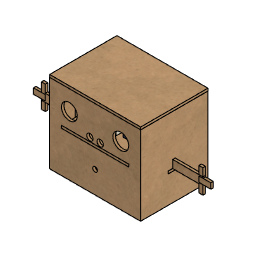
CAD final (Autodesk Fusion 360 design; units mm, degrees)
Autodesk Fusion 360 part; units mm, degrees
sketch "Sketch1" plane through (0, 0, 0) normal (0, 0, 1) x (1, 0, 0)
  line L0 (-32.3795, 47.4843) -> (40, 47.4843)
  line L1 (40, 47.4843) -> (40, -5)
  line L2 (40, -5) -> (-32.3795, -5)
  line L3 (-32.3795, -5) -> (-32.3795, 47.4843)
  constraint horizontal L0
  constraint vertical L1
  constraint horizontal L2
  constraint vertical L3
sketch "Sketch2" plane through (0, 0, 0) normal (0, 0, 1) x (1, 0, 0)
sketch "Sketch3" plane through (0, 0, 0) normal (0, 0, 1) x (1, 0, 0)
  line L0 (-70, 30) -> (-16.7, 30)
  line L1 (-16.7, 30) -> (-16.7, -38.6)
  line L2 (-16.7, -38.6) -> (-70, -38.6)
  line L3 (-70, -38.6) -> (-70, 30)
  dimension "d3" = 53.3
  dimension "d4" = 68.6
  constraint horizontal L0
  constraint vertical L1
  constraint horizontal L2
  constraint vertical L3
  measures "d3" distance of L0.start L0.end
  measures "d4" distance of L0.start L2.end
extrude "Extrude2" add sketch "Sketch3" along normal blind 10 makes body 1
move_body "Move3" bodies 1 to x (0, -1, 0) y (1, 0, 0) z (0, 0, 1) at (-31.4, -108.6, 0)
move_body "Move4" bodies 1 to x (1, 0, 0) y (0, 1, 0) z (0, 0, 1) at (-5.9347, 58.8273, -1.6422)
sketch "Sketch4" plane through (0, 0, 0) normal (0, 0, 1) x (1, 0, 0)
  line L0 (40, 25) -> (125, 25)
  line L1 (125, 25) -> (125, -30)
  line L2 (125, -30) -> (40, -30)
  line L3 (40, -30) -> (40, 25)
  dimension "d7" = 85
  dimension "d8" = 55
  constraint horizontal L0
  constraint vertical L1
  constraint horizontal L2
  constraint vertical L3
  measures "d7" distance of L0.start L0.end
  measures "d8" distance of L0.start L2.end
extrude "Extrude3" add sketch "Sketch4" along normal blind 10 separate body makes body 2
move_body "Move5" bodies 1 to x (0, 1, 0) y (-1, 0, 0) z (0, 0, 1) at (-109.0073, 42.862, 0)
move_body "Move6" bodies 1 to x (1, 0, 0) y (0, 1, 0) z (0, 0, 1) at (69.2901, 3.0727, 11.6422)
move_body "Move7" bodies 2 to x (0, 1, 0) y (-1, 0, 0) z (0, 0, 1) at (10, -70, 0)
move_body "Move8" bodies 2 to x (1, 0, 0) y (0, 1, 0) z (0, 0, 1) at (13.4816, 0.9657, 8.7354)
sketch "Sketch5" plane through (0, 0, 0) normal (0, 0, 1) x (1, 0, 0)
  line L0 (100, -150) -> (-130, -150)
  line L1 (-130, -150) -> (-130, 20)
  line L2 (-130, 20) -> (100, 20)
  line L3 (100, 20) -> (100, -150)
  dimension "d11" = 230
  dimension "d12" = 170
  constraint horizontal L0
  constraint vertical L1
  constraint horizontal L2
  constraint vertical L3
  measures "d11" distance of L0.start L0.end
  measures "d12" distance of L0.start L2.end
extrude "Extrude4" add sketch "Sketch5" against normal blind 200 separate body makes body 3
sketch "Sketch6" plane through (0, 0, -200) normal (0, 0, -1) x (1, 0, 0)
  line L0 (-130, -20) -> (100, -20)
  line L1 (100, -20) -> (100, 150)
  line L2 (100, 150) -> (-130, 150)
  line L3 (-130, 150) -> (-130, -20)
  line L4 (-122.8889, 140.963) -> (94.4111, 140.963)
  line L5 (94.4111, 140.963) -> (94.4111, -12.737)
  line L6 (94.4111, -12.737) -> (-122.8889, -12.737)
  line L7 (-122.8889, -12.737) -> (-122.8889, 140.963)
  dimension "d15" = 217.3
  dimension "d16" = 153.7
  constraint horizontal L4
  constraint vertical L5
  constraint horizontal L6
  constraint vertical L7
  measures "d15" distance of L4.start L4.end
  measures "d16" distance of L4.start L6.end
extrude "Extrude5" cut sketch "Sketch6" against normal blind 193.35 contours L4 L5 L6 L7 bodies 3
move_body "Move9" bodies 1 to x (1, 0, 0) y (0, 1, 0) z (0, 0, 1) at (-192.1553, -38.6436, -133.7239)
move_body "Move10" bodies 2 to x (1, 0, 0) y (0, 1, 0) z (0, 0, 1) at (-190.1426, -42.9302, -139.0807)
sketch "Sketch7" plane through (0, 0, 0) normal (0, 0, 1) x (1, 0, 0)
  line L0 (-116.7221, 87.5547) -> (113.2779, 87.5547)
  line L1 (113.2779, 87.5547) -> (113.2779, 257.5547)
  line L2 (113.2779, 257.5547) -> (-116.7221, 257.5547)
  line L3 (-116.7221, 257.5547) -> (-116.7221, 87.5547)
  dimension "d19" = 230
  dimension "d20" = 170
  constraint horizontal L0
  constraint vertical L1
  constraint horizontal L2
  constraint vertical L3
  measures "d19" distance of L0.start L0.end
  measures "d20" distance of L0.start L2.end
extrude "Extrude6" add sketch "Sketch7" along normal blind 6.35 separate body makes body 4
move_body "Move11" bodies 4 to x (1, 0, 0) y (0, 1, 0) z (0, 0, 1) at (-13.2084, -237.8923, -206.1761)
sketch "Sketch8" plane through (0, 20, 0) normal (0, 1, 0) x (-1, 0, 0)
  line L0 (130, 0) -> (-100, 0)
  line L1 (-100, 0) -> (-100, -200)
  line L2 (-100, -200) -> (130, -200)
  line L3 (130, -200) -> (130, 0)
  line L4 (100, -110) -> (-72.7396, -110)
  line L5 (-72.7396, -110) -> (-72.7396, -103.65)
  line L6 (-72.7396, -103.65) -> (100, -103.65)
  line L7 (100, -103.65) -> (100, -110)
  dimension "d23" = 6.35
  constraint horizontal L4
  constraint vertical L5
  constraint horizontal L6
  constraint vertical L7
  measures "d23" distance of L4.start L6.end
extrude "Extrude7" cut sketch "Sketch8" against normal blind 200 contours L4 L5 L6 L7 bodies 3
sketch "Sketch9" plane through (0, 0, 0) normal (0, 0, 1) x (1, 0, 0)
  line L0 (-120, 110) -> (52.74, 110)
  line L1 (52.74, 110) -> (52.74, 280)
  line L2 (52.74, 280) -> (-120, 280)
  line L3 (-120, 280) -> (-120, 110)
  dimension "d26" = 172.74
  dimension "d27" = 170
  constraint horizontal L0
  constraint vertical L1
  constraint horizontal L2
  constraint vertical L3
  measures "d26" distance of L0.start L0.end
  measures "d27" distance of L0.start L2.end
extrude "Extrude8" add sketch "Sketch9" against normal blind 6.35 separate body makes body 5
move_body "Move12" bodies 5 to x (1, 0, 0) y (0, 1, 0) z (0, 0, 1) at (20.107, -259.5032, -103.2368)
sketch "Sketch10" plane through (0, -150, 0) normal (0, -1, 0) x (1, 0, 0)
  line L0 (72.7396, -103.65) -> (72.7396, -110)
  line L1 (72.7396, -110) -> (-100, -110)
  line L2 (-100, -110) -> (-100, -103.65)
  line L3 (-100, -103.65) -> (72.7396, -103.65)
  line L4 (100, 0) -> (-130, 0)
  line L5 (-130, 0) -> (-130, -200)
  line L6 (-130, -200) -> (100, -200)
  line L7 (100, -200) -> (100, 0)
  circle A0 centre (50, -150) radius 20
  circle A1 centre (50, -150) radius 20
  circle A2 centre (-80, -150) radius 20
extrude "Extrude9" cut sketch "Sketch10" against normal blind 20 contours A0 A1 | A2 bodies 3
sketch "Sketch11" plane through (0, -150, 0) normal (0, -1, 0) x (1, 0, 0)
  circle A0 centre (-80, -150) radius 20
  circle A1 centre (50, -150) radius 20
  line L0 (72.7396, -103.65) -> (72.7396, -110)
  line L1 (72.7396, -110) -> (-100, -110)
  line L2 (-100, -110) -> (-100, -103.65)
  line L3 (-100, -103.65) -> (72.7396, -103.65)
  line L4 (100, 0) -> (-130, 0)
  line L5 (-130, 0) -> (-130, -200)
  line L6 (-130, -200) -> (100, -200)
  line L7 (100, -200) -> (100, 0)
  circle A2 centre (-1.9497, -120.0498) radius 8.05
  dimension "d32" = 16.1
  measures "d32" diameter of A2
sketch "Sketch12" plane through (0, -150, 0) normal (0, -1, 0) x (1, 0, 0)
sketch "Sketch13" plane through (0, -150, 0) normal (0, -1, 0) x (1, 0, 0)
  circle A0 centre (-28.05, -120.05) radius 8.05
  dimension "d33" = 16.1
  measures "d33" diameter of A0
extrude "Extrude10" cut sketch "Sketch11" sketch "Sketch13" against normal blind 10 contours A2 of sketch 2 bodies 3
move_body "Move13" bodies 4 to x (1, 0, 0) y (0, 1, 0) z (0, 0, 1) at (231.7541, -19.2478, 6.1761)
move_body "Move14" bodies 2 to x (1, 0, 0) y (0, 1, 0) z (0, 0, 1) at (189.899, -32.0286, 10.5679)
move_body "Move15" bodies 1 to x (1, 0, 0) y (0, 1, 0) z (0, 0, 1) at (183.6878, -30.6758, -12.2886)
move_body "Move16" bodies 1 to x (1, 0, 0) y (0, 1, 0) z (0, 0, 1) at (0, 0, 15)
sketch "Sketch14" plane through (100, 0, 0) normal (1, 0, 0) x (0, 1, 0)
sketch "Sketch15" plane through (100, 0, 0) normal (1, 0, 0) x (0, 1, 0)
  line L0 (-50, -75) -> (-80, -75)
  line L1 (-80, -75) -> (-80, -68.65)
  line L2 (-80, -68.65) -> (-50, -68.65)
  line L3 (-50, -68.65) -> (-50, -75)
  dimension "d36" = 6.35
  constraint horizontal L0
  constraint vertical L1
  constraint horizontal L2
  constraint vertical L3
  measures "d36" distance of L0.start L2.end
extrude "Extrude11" cut sketch "Sketch15" against normal blind 320 bodies 3
sketch "Sketch16" plane through (0, 0, 0) normal (0, 0, 1) x (1, 0, 0)
  line L0 (-100, 140) -> (130, 140)
  line L1 (130, 140) -> (130, 170)
  line L2 (130, 170) -> (-100, 170)
  line L3 (-100, 170) -> (-100, 140)
  dimension "d39" = 230
  dimension "d40" = 30
  constraint horizontal L0
  constraint vertical L1
  constraint horizontal L2
  constraint vertical L3
  measures "d39" distance of L0.start L0.end
  measures "d40" distance of L0.start L2.end
extrude "Extrude12" add sketch "Sketch16" against normal blind 6.35 separate body makes body 6
move_body "Move17" bodies 6 to x (1, 0, 0) y (0, 1, 0) z (0, 0, 1) at (-29.7399, -217.8653, -68.3754)
move_body "Move18" bodies 6 to x (1, 0, 0) y (0, 1, 0) z (0, 0, 1) at (0, -2.152, 0)
sketch "Sketch17" plane through (0, 0, -74.7254) normal (0, 0, -1) x (1, 0, 0)
  line L0 (-129.7399, 80.0173) -> (-129.7399, 50.0173)
  line L1 (-129.7399, 50.0173) -> (100.2601, 50.0173)
  line L2 (100.2601, 50.0173) -> (100.2601, 80.0173)
  line L3 (100.2601, 80.0173) -> (-129.7399, 80.0173)
sketch "Sketch18" plane through (0, 0, -74.7254) normal (0, 0, -1) x (1, 0, 0)
  line L0 (90.26, 76.717) -> (86.61, 76.717)
  line L1 (86.61, 76.717) -> (86.61, 64.717)
  line L2 (86.61, 64.717) -> (90.26, 64.717)
  line L3 (90.26, 64.717) -> (90.26, 76.717)
  dimension "d43" = 3.65
  constraint horizontal L0
  constraint vertical L1
  constraint horizontal L2
  constraint vertical L3
  measures "d43" distance of L0.start L0.end
sketch "Sketch19" plane through (0, 0, -74.7254) normal (0, 0, -1) x (1, 0, 0)
  line L0 (60.61, 64.717) -> (56.96, 64.717)
  line L1 (56.96, 64.717) -> (56.96, 76.717)
  line L2 (56.96, 76.717) -> (60.61, 76.717)
  line L3 (60.61, 76.717) -> (60.61, 64.717)
  dimension "d44" = 3.65
  constraint horizontal L0
  constraint vertical L1
  constraint horizontal L2
  constraint vertical L3
  measures "d44" distance of L0.start L0.end
extrude "Extrude13" cut sketch "Sketch18" against normal blind 11 bodies 6
extrude "Extrude14" cut sketch "Sketch19" against normal blind 22 bodies 6
sketch "Sketch20" plane through (0, 0, 0) normal (0, 0, 1) x (1, 0, 0)
  line L0 (95, -105) -> (91.35, -105)
  line L1 (91.35, -105) -> (91.35, -117)
  line L2 (91.35, -117) -> (95, -117)
  line L3 (95, -117) -> (95, -105)
  dimension "d49" = 3.65
  dimension "d50" = 12
  constraint horizontal L0
  constraint vertical L1
  constraint horizontal L2
  constraint vertical L3
  measures "d49" distance of L0.start L0.end
  measures "d50" distance of L0.start L2.end
sketch "Sketch21" plane through (0, 0, 0) normal (0, 0, 1) x (1, 0, 0)
  line L0 (65.35, -105) -> (61.7, -105)
  line L1 (61.7, -105) -> (61.7, -117)
  line L2 (61.7, -117) -> (65.35, -117)
  line L3 (65.35, -117) -> (65.35, -105)
  dimension "d51" = 3.65
  dimension "d52" = 12
  constraint horizontal L0
  constraint vertical L1
  constraint horizontal L2
  constraint vertical L3
  measures "d51" distance of L0.start L0.end
  measures "d52" distance of L0.start L2.end
extrude "Extrude15" add sketch "Sketch21" against normal blind 25 separate body makes body 7
extrude "Extrude16" add sketch "Sketch20" against normal blind 25 separate body makes body 8
extrude "Extrude17" cut 1 faces at (86.61, -72.717, -72.6087) along direction (-1, 0, 0) blind 2.65 on bodies 6 bodies 6
extrude "Extrude18" cut 1 faces at (83.96, -72.717, -72.6087) along direction (-1, 0, 0) blind 0.05 on bodies 6 bodies 6
extrude "Extrude19" cut 1 faces at (56.96, -68.717, -72.6087) along direction (-1, 0, 0) blind 6.35 on bodies 6 bodies 6
extrude "Extrude20" add 1 faces at (60.61, -72.717, -72.6087) along direction (-1, 0, 0) blind 3.3 on bodies 6 bodies 6
extrude "Extrude21" cut 1 faces at (57.31, -72.717, -72.6087) along direction (1, 0, 0) blind 0.6 on bodies 6 bodies 6
extrude "Extrude22" add 1 faces at (50.61, -68.717, -72.6087) along direction (1, 0, 0) blind 0.95 on bodies 6 bodies 6
extrude "Extrude23" add 1 faces at (91.35, -109, -8.3333) along direction (-1, 0, 0) blind 0.7 on bodies 8 bodies 8
extrude "Extrude24" cut 1 faces at (65.35, -113, -8.3333) along direction (-1, 0, 0) blind 0.7 on bodies 7 bodies 7
extrude "Extrude25" add 1 faces at (61.7, -109, -8.3333) along direction (-1, 0, 0) blind 1.4 on bodies 7 bodies 7
extrude "Extrude26" add 1 faces at (90.65, -109, -8.3333) along direction (-1, 0, 0) blind 2 on bodies 8 bodies 8
extrude "Extrude27" cut 1 faces at (64.65, -113, -8.3333) along direction (-1, 0, 0) blind 2 on bodies 7 bodies 7
extrude "Extrude28" add 1 faces at (60.3, -109, -8.3333) along direction (-1, 0, 0) blind 4 on bodies 7 bodies 7
sketch "Sketch22" plane through (56.3, 0, 0) normal (-1, 0, 0) x (0, -1, 0)
extrude "Extrude29" cut 1 faces at (86.0267, -64.717, -70.4921) along direction (0, 1, 0) blind 10 on bodies 6 bodies 6
extrude "Extrude30" cut 1 faces at (53.6767, -64.717, -70.4921) along direction (0, 1, 0) blind 10 on bodies 6 bodies 6
extrude "Extrude31" add 1 faces at (60.5333, -105, -8.3333) along direction (0, 1, 0) blind 10 on bodies 7 bodies 7
extrude "Extrude32" add 1 faces at (92.8833, -105, -8.3333) along direction (0, 1, 0) blind 10 on bodies 8 bodies 8
sketch "Sketch23" plane through (56.3, 0, 0) normal (-1, 0, 0) x (0, -1, 0)
  line L0 (113.4998, -12.7498) -> (98.4998, -12.7498)
  line L1 (98.4998, -12.7498) -> (98.4998, -6.3998)
  line L2 (98.4998, -6.3998) -> (113.4998, -6.3998)
  line L3 (113.4998, -6.3998) -> (113.4998, -12.7498)
  dimension "d91" = 15
  dimension "d92" = 6.35
  constraint horizontal L0
  constraint vertical L1
  constraint horizontal L2
  constraint vertical L3
  measures "d91" distance of L0.start L0.end
  measures "d92" distance of L0.start L2.end
extrude "Extrude33" add 1 faces at (60.5333, -109.6667, -25) along direction (0, 0, -1) blind 5.85 on bodies 7 bodies 7
extrude "Extrude34" add 1 faces at (90.7667, -102.3333, -25) along direction (0, 0, -1) blind 5.85 on bodies 8 bodies 8
sketch "Sketch24" plane through (56.3, 0, 0) normal (-1, 0, 0) x (0, -1, 0)
  line L0 (95, -30.85) -> (117, -30.85)
  line L1 (113.5, -31) -> (98.5, -31)
  line L2 (98.5, -31) -> (98.5, -24.65)
  line L3 (98.5, -24.65) -> (113.5, -24.65)
  line L4 (113.5, -24.65) -> (113.5, -31)
  dimension "d97" = 15
  dimension "d98" = 6.35
  constraint horizontal L1
  constraint vertical L2
  constraint horizontal L3
  constraint vertical L4
  measures "d97" distance of L1.start L1.end
  measures "d98" distance of L1.start L3.end
extrude "Extrude35" add 1 faces at (60.5333, -109.6667, -30.85) along direction (0, 0, -1) blind 3 on bodies 7 bodies 7
extrude "Extrude36" add 1 faces at (90.7667, -102.3333, -30.85) along direction (0, 0, -1) blind 3 on bodies 8 bodies 8
extrude "Extrude37" cut sketch "Sketch24" against normal blind 41 contours L0 L2 L3 L4 bodies 7 8
extrude "Extrude38" cut sketch "Sketch23" against normal blind 39 bodies 7 8
sketch "Sketch25" plane through (0, 0, 0) normal (0, 0, 1) x (1, 0, 0)
  line L0 (55, -135) -> (93.7, -135)
  line L1 (93.7, -135) -> (93.7, -150)
  line L2 (93.7, -150) -> (55, -150)
  line L3 (55, -150) -> (55, -135)
  dimension "d107" = 38.7
  constraint horizontal L0
  constraint vertical L1
  constraint horizontal L2
  constraint vertical L3
  measures "d107" distance of L0.start L0.end
extrude "Extrude39" add sketch "Sketch25" along normal blind 6.35 separate body makes body 9
move_body "Move19" bodies 9 to x (1, 0, 0) y (0, 1, 0) z (0, 0, 1) at (1.3032, 36.5589, -12.7529)
sketch "Sketch26" plane through (0, 0, 0) normal (0, 0, 1) x (1, 0, 0)
  line L0 (-30, 12) -> (8.7, 12)
  line L1 (8.7, 12) -> (8.7, -3)
  line L2 (8.7, -3) -> (-30, -3)
  line L3 (-30, -3) -> (-30, 12)
  dimension "d110" = 38.7
  dimension "d111" = 15
  constraint horizontal L0
  constraint vertical L1
  constraint horizontal L2
  constraint vertical L3
  measures "d110" distance of L0.start L0.end
  measures "d111" distance of L0.start L2.end
extrude "Extrude40" add sketch "Sketch26" along normal blind 6.35 separate body makes body 10
move_body "Move20" bodies 10 to x (1, 0, 0) y (0, 1, 0) z (0, 0, 1) at (86.3471, -110.4772, -31.0644)
move_body "Move21" bodies 7 8 9 10 to x (1, 0, 0) y (0, 1, 0) z (0, 0, 1) at (-4.8384, 40.4721, -68.412)
move_body "Move22" bodies 4 to x (1, 0, 0) y (0, 1, 0) z (0, 0, 1) at (-231.998, 19.5704, 0)
sketch "Sketch27" plane through (94.4111, 0, 0) normal (-1, 0, 0) x (0, -1, 0)
  line L0 (80, -68.65) -> (80, -75)
  line L1 (80, -75) -> (50, -75)
  line L2 (50, -75) -> (50, -68.65)
  line L3 (50, -68.65) -> (80, -68.65)
  line L4 (-12.737, -200) -> (140.963, -200)
  line L5 (140.963, -200) -> (140.963, -6.65)
  line L6 (140.963, -6.65) -> (-12.737, -6.65)
  line L7 (-12.737, -6.65) -> (-12.737, -200)
  line L8 (95, -75) -> (88.65, -75)
  line L9 (88.65, -75) -> (88.65, -111.7682)
  line L10 (88.65, -111.7682) -> (95, -111.7682)
  line L11 (95, -111.7682) -> (95, -75)
  dimension "d114" = 6.35
  constraint horizontal L8
  constraint vertical L9
  constraint horizontal L10
  constraint vertical L11
  measures "d114" distance of L8.start L8.end
extrude "Extrude41" add 1 faces at (72.7396, -143.9753, -107.8833) along direction (-1, 0, 0) blind 2.74 on bodies 3 bodies 3
extrude "Extrude42" cut 1 faces at (72.847, -92.8366, -105.3534) along direction (-1, 0, 0) blind 2.74 on bodies 5 bodies 5
move_body "Move23" bodies 5 to x (1, 0, 0) y (0, 1, 0) z (0, 0, 1) at (0.1843, 0, -0.3685)
extrude "Extrude43" add 1 faces at (72.7396, 17.579, -107.8833) along direction (-1, 0, 0) blind 2.74 on bodies 3 bodies 3
extrude "Extrude44" cut sketch "Sketch27" against normal blind 15 contours L8 L9 L10 L11 bodies 3
extrude "Extrude45" cut 1 faces at (98.137, -90.7667, -111.7682) along direction (0, 0, -1) blind 28 on bodies 3 bodies 3
extrude "Extrude46" cut 1 faces at (96.2741, -95, -118.1788) along direction (0, -1, 0) blind 1.5 on bodies 3 bodies 3
sketch "Sketch28" plane through (0, 0, 0) normal (0, 0, 1) x (1, 0, 0)
  line L0 (60, 60) -> (180, 60)
  line L1 (180, 60) -> (180, 80)
  line L2 (180, 80) -> (60, 80)
  line L3 (60, 80) -> (60, 60)
  constraint horizontal L0
  constraint vertical L1
  constraint horizontal L2
  constraint vertical L3
extrude "Extrude47" add sketch "Sketch28" along normal blind 6.35 separate body makes body 11
extrude "Extrude48" add 1 faces at (94.4111, -8.1753, -93.8833) along direction (-1, 0, 0) blind 0.761 on bodies 3 bodies 3 7 8 9 10 6
extrude "Extrude49" cut 1 faces at (13.5869, -140.963, -38.9833) along direction (0, -1, 0) blind 2.687 on bodies 3 bodies 3
extrude "Extrude50" cut 1 faces at (-122.8889, -70.3043, -158.3333) along direction (-1, 0, 0) blind 0.761 on bodies 3 bodies 3
extrude "Extrude51" cut 1 faces at (13.3333, 12.737, -38.9833) along direction (0, 1, 0) blind 0.913 on bodies 3 bodies 3
sketch "Sketch29" plane through (0, 0, 0) normal (0, 0, 1) x (1, 0, 0)
  line L0 (175, 45) -> (205, 45)
  line L1 (205, 45) -> (205, 55)
  line L2 (205, 55) -> (175, 55)
  line L3 (175, 55) -> (175, 45)
  dimension "d139" = 30
  dimension "d140" = 10
  constraint horizontal L0
  constraint vertical L1
  constraint horizontal L2
  constraint vertical L3
  measures "d139" distance of L0.start L0.end
  measures "d140" distance of L0.start L2.end
extrude "Extrude52" add sketch "Sketch29" along normal blind 6.35 separate body makes body 12
move_body "Move24" bodies 12 to x (0.642788, -0.766044, 0) y (0.766044, 0.642788, 0) z (0, 0, 1) at (20.3326, 165.0215, 1.3134)
move_body "Move25" bodies 12 to x (1, 0, 0) y (0, 1, 0) z (0, 0, 1) at (0, 0, -1)
move_body "Move26" bodies 12 to x (1, 0, 0) y (0, 1, 0) z (0, 0, 1) at (0, 0, -0.31)
move_body "Move27" bodies 12 to x (0.766044, -0.642788, 0) y (0.642788, 0.766044, 0) z (0, 0, 1) at (15.4151, 116.1683, 0)
move_body "Move28" bodies 12 to x (1, 0, 0) y (0, 1, 0) z (0, 0, 1) at (-12, 7, 0)
move_body "Move29" bodies 12 to x (1, 0, 0) y (0, 1, 0) z (0, 0, 1) at (-0.065, 0, 0)
move_body "Move30" bodies 12 to x (1, 0, 0) y (0, 1, 0) z (0, 0, 1) at (0, 8.487, 0)
sketch "Sketch30" plane through (0, 0, 0) normal (0, 0, 1) x (1, 0, 0)
  line L0 (158.5541, 93.3276) -> (188.5541, 93.3276)
  line L1 (188.5541, 93.3276) -> (188.5541, 103.3276)
  line L2 (188.5541, 103.3276) -> (158.5541, 103.3276)
  line L3 (158.5541, 103.3276) -> (158.5541, 93.3276)
  dimension "d143" = 30
  dimension "d144" = 10
  constraint horizontal L0
  constraint vertical L1
  constraint horizontal L2
  constraint vertical L3
  measures "d143" distance of L0.start L0.end
  measures "d144" distance of L0.start L2.end
extrude "Extrude53" add sketch "Sketch30" along normal blind 6.35 separate body makes body 13
move_body "Move31" bodies 13 to x (0, 1, 0) y (-1, 0, 0) z (0, 0, 1) at (272.8817, -79.2265, 0)
move_body "Move32" bodies 13 to x (1, 0, 0) y (0, 1, 0) z (0, 0, 1) at (0.446, 0, 0)
move_body "Move33" bodies 13 to x (1, 0, 0) y (0, 1, 0) z (0, 0, 1) at (0, -9.328, 0)
sketch "Sketch31" plane through (0, 0, 0) normal (0, 0, 1) x (1, 0, 0)
  line L0 (185, 65) -> (215, 65)
  line L1 (215, 65) -> (215, 75)
  line L2 (215, 75) -> (185, 75)
  line L3 (185, 75) -> (185, 65)
  dimension "d147" = 30
  dimension "d148" = 10
  constraint horizontal L0
  constraint vertical L1
  constraint horizontal L2
  constraint vertical L3
  measures "d147" distance of L0.start L0.end
  measures "d148" distance of L0.start L2.end
extrude "Extrude54" add sketch "Sketch31" along normal blind 6.35 separate body makes body 14
move_body "Move34" bodies 14 to x (1, 0, 0) y (0, 1, 0) z (0, 0, 1) at (-12.5051, 0.0024, -0.0344)
move_face "MoveFace1" by (0, 0.002, 0) 1 faces at (182.4949, 71.6691, -0.0344) on bodies 14
move_body "Move35" bodies 14 to x (1, 0, 0) y (0, 1, 0) z (0, 0, 1) at (0, 0.002, 0)
move_body "Move36" bodies 14 to x (1, 0, 0) y (0, 1, 0) z (0, 0, 1) at (-2.495, 0, 0)
move_body "Move37" bodies 11 14 12 13 to x (1, 0, 0) y (0, 0, -1) z (0, 1, 0) at (0, -95.7396, -20.3656)
extrude "Extrude55" add 1 faces at (179.9999, -93.6574, -85.37) along direction (0, 0, 1) blind 2 on bodies 14 bodies 14 13 11 12
extrude "Extrude56" add 1 faces at (193.3333, -93.6459, -95.37) along direction (0, 0, -1) blind 2 on bodies 14 bodies 14 13
extrude "Extrude57" cut 1 faces at (95.7667, -88.65, -118.1788) along direction (0, 1, 0) blind 5 on bodies 3 bodies 3
move_body "Move38" bodies 14 to x (1, 0, 0) y (0, 1, 0) z (0, 0, 1) at (0, 5, 0)
extrude "Extrude58" add 1 faces at (97.8834, -96.5, -118.1788) along direction (0, 1, 0) blind 5 on bodies 3 bodies 3
move_body "Move39" bodies 1 to x (1, 0, 0) y (0, 1, 0) z (0, 0, 1) at (-20, 0, 0)
move_body "Move40" bodies 2 to x (1, 0, 0) y (0, 1, 0) z (0, 0, 1) at (-20, 0, 0)
sketch "Sketch32" plane through (0, 0, -109.9553) normal (0, 0, -1) x (1, 0, 0)
  line L0 (70.2912, -20.4968) -> (70.2912, 149.5032)
  line L1 (70.2912, 149.5032) -> (-99.7088, 149.5032)
  line L2 (-99.7088, 149.5032) -> (-99.7088, -20.4968)
  line L3 (-99.7088, -20.4968) -> (70.2912, -20.4968)
  line L4 (70.2912, 83.9013) -> (45.1656, 83.9013)
  line L5 (45.1656, 83.9013) -> (45.1656, 90.3613)
  line L6 (45.1656, 90.3613) -> (70.2912, 90.3613)
  line L7 (70.2912, 90.3613) -> (70.2912, 83.9013)
  dimension "d159" = 6.46
  constraint horizontal L4
  constraint vertical L5
  constraint horizontal L6
  constraint vertical L7
  constraint coincident L0 L4.start
  measures "d159" distance of L4.start L6.end
extrude "Extrude59" cut sketch "Sketch32" against normal blind 7 contours L0 L4 L5 L6 L7 bodies 5
extrude "Extrude60" cut 1 faces at (53.5408, -90.3613, -107.8386) along direction (0, -1, 0) blind 1 on bodies 5 bodies 5
sketch "Sketch33" plane through (0, -150, 0) normal (0, -1, 0) x (1, 0, 0)
  circle A0 centre (-1.9497, -120.0498) radius 8.05
  circle A1 centre (-28.05, -120.05) radius 8.05
  circle A2 centre (-80, -150) radius 20
  circle A3 centre (50, -150) radius 20
  line L0 (69.9996, -103.65) -> (69.9996, -110)
  line L1 (69.9996, -110) -> (-100, -110)
  line L2 (-100, -110) -> (-100, -103.65)
  line L3 (-100, -103.65) -> (69.9996, -103.65)
  line L4 (100, 0) -> (-130, 0)
  line L5 (-130, 0) -> (-130, -200)
  line L6 (-130, -200) -> (100, -200)
  line L7 (100, -200) -> (100, 0)
  circle A4 centre (-15.0002, -56.1498) radius 17.5
  dimension "d164" = 35
  measures "d164" diameter of A4
extrude "Extrude61" cut sketch "Sketch33" against normal blind 15 contours A4 bodies 3
copy_body "CopyPasteBodies1" bodies 14 makes body 15
move_body "Move41" bodies 15 to x (-1, 0, 0) y (0, 1, 0) z (0, 0, -1) at (-145.6101, 24.6968, -200.2325)
combine "Combine1" operation add target body 7 tool bodies 8 10 9
sketch "Sketch34" plane through (0, 0, -74.7254) normal (0, 0, -1) x (1, 0, 0)
  line L0 (90.26, 76.717) -> (90.26, 54.717)
  line L1 (90.26, 54.717) -> (83.91, 54.717)
  line L2 (83.91, 54.717) -> (83.91, 76.717)
  line L3 (83.91, 76.717) -> (90.26, 76.717)
  line L4 (100, 80.0173) -> (100, 80)
  line L5 (100, 80) -> (93.6501, 80)
  line L6 (93.6501, 80) -> (93.6501, 80.0173)
  line L7 (93.6501, 80.0173) -> (-123.6499, 80.0173)
  line L8 (-123.6499, 80.0173) -> (-123.6499, 80)
  line L9 (-123.6499, 80) -> (-129.7399, 80)
  line L10 (-129.7399, 80) -> (-129.7399, 50.0173)
  line L11 (-129.7399, 50.0173) -> (100.2601, 50.0173)
  line L12 (100.2601, 50.0173) -> (100.2601, 80.0173)
  line L13 (100.2601, 80.0173) -> (100, 80.0173)
  line L14 (51.56, 54.717) -> (51.56, 76.717)
  line L15 (51.56, 76.717) -> (57.91, 76.717)
  line L16 (57.91, 76.717) -> (57.91, 54.717)
  line L17 (57.91, 54.717) -> (51.56, 54.717)
  line L18 (-118.1992, 75.6846) -> (-111.8492, 75.6846)
  line L19 (-111.8492, 75.6846) -> (-111.8492, 53.6846)
  line L20 (-111.8492, 53.6846) -> (-118.1992, 53.6846)
  line L21 (-118.1992, 53.6846) -> (-118.1992, 75.6846)
  line L22 (-85.8496, 54.619) -> (-85.8496, 76.619)
  line L23 (-85.8496, 76.619) -> (-79.4996, 76.619)
  line L24 (-79.4996, 76.619) -> (-79.4996, 54.619)
  line L25 (-79.4996, 54.619) -> (-85.8496, 54.619)
  dimension "d167" = 6.35
  dimension "d168" = 22
  dimension "d169" = 6.35
  dimension "d170" = 22
  constraint horizontal L18
  constraint vertical L19
  constraint horizontal L20
  constraint vertical L21
  constraint horizontal L23
  constraint vertical L24
  constraint horizontal L25
  constraint vertical L22
  measures "d167" distance of L18.start L18.end
  measures "d168" distance of L18.start L20.end
  measures "d169" distance of L22.end L23.end
  measures "d170" distance of L22.end L22.start
extrude "Extrude62" cut sketch "Sketch34" against normal blind 9 contours L18 L19 L20 L21 | L22 L23 L24 L25 bodies 3
sketch "Sketch35" plane through (0, 0, 0) normal (0, 0, 1) x (1, 0, 0)
  line L0 (-140, 50) -> (-133.65, 50)
  line L1 (-133.65, 50) -> (-133.65, 72)
  line L2 (-133.65, 72) -> (-140, 72)
  line L3 (-140, 72) -> (-140, 50)
  line L4 (-107.65, 72) -> (-107.65, 50)
  line L5 (-107.65, 50) -> (-101.3, 50)
  line L6 (-101.3, 50) -> (-101.3, 72)
  line L7 (-101.3, 72) -> (-107.65, 72)
  dimension "d173" = 6.35
  dimension "d174" = 22
  dimension "d175" = 6.35
  dimension "d176" = 22
  constraint horizontal L0
  constraint vertical L1
  constraint horizontal L2
  constraint vertical L3
  constraint horizontal L5
  constraint vertical L6
  constraint horizontal L7
  constraint vertical L4
  measures "d173" distance of L0.start L0.end
  measures "d174" distance of L0.start L2.end
  measures "d175" distance of L4.end L5.end
  measures "d176" distance of L4.end L4.start
extrude "Extrude63" add sketch "Sketch35" against normal blind 25 separate body makes body 16 at (-140, 64.6667, -8.3333) makes body 17 at (-101.3, 57.3333, -8.3333)
extrude "Extrude64" add 2 faces at (-105.5333, 64.6667, -25) (-137.8833, 64.6667, -25) along direction (0, 0, -1) blind 8.85 on bodies 16 17 bodies 17 16
sketch "Sketch36" plane through (-101.3, 0, 0) normal (1, 0, 0) x (0, 1, 0)
  line L0 (72, 0) -> (50, 0)
  line L1 (50, 0) -> (50, -33.85)
  line L2 (50, -33.85) -> (72, -33.85)
  line L3 (72, -33.85) -> (72, 0)
  line L4 (64.18, -29) -> (57.82, -29)
  line L5 (57.82, -29) -> (57.82, -9)
  line L6 (57.82, -9) -> (64.18, -9)
  line L7 (64.18, -9) -> (64.18, -29)
  dimension "d181" = 6.36
  dimension "d182" = 20
  constraint horizontal L4
  constraint vertical L5
  constraint horizontal L6
  constraint vertical L7
  measures "d181" distance of L4.start L4.end
  measures "d182" distance of L4.start L6.end
extrude "Extrude65" cut sketch "Sketch36" against normal blind 5 contours L4 L5 L6 L7 bodies 17
move_body "Move42" bodies 17 16 to x (1, 0, 0) y (0, 1, 0) z (0, 0, 1) at (21.914, -126.6086, -68.2792)
move_body "Move43" bodies 16 to x (1, 0, 0) y (0, 1, 0) z (0, 0, 1) at (0, 1, 0)
move_body "Move44" bodies 16 17 to x (1, 0, 0) y (0, 1, 0) z (0, 0, 1) at (0, 0, 2)
move_body "Move45" bodies 17 16 to x (1, 0, 0) y (0, 1, 0) z (0, 0, 1) at (0, 0, 0.565)
move_body "Move46" bodies 16 17 to x (1, 0, 0) y (0, 1, 0) z (0, 0, 1) at (0, 0, -0.6)
move_body "Move47" bodies 17 to x (1, 0, 0) y (0, 1, 0) z (0, 0, 1) at (0, 0, -20)
extrude "Extrude66" cut 1 faces at (-85.8496, -61.9524, -72.6087) along direction (-1, 0, 0) blind 15 on bodies 3 bodies 3
extrude "Extrude67" add 1 faces at (-79.4996, -69.2857, -72.6087) along direction (-1, 0, 0) blind 15 on bodies 3 bodies 3
move_body "Move48" bodies 17 to x (1, 0, 0) y (0, 1, 0) z (0, 0, 1) at (-15, 0, 0)
move_body "Move49" bodies 17 to x (1, 0, 0) y (0, 1, 0) z (0, 0, 1) at (0, 0, 20)
extrude "Extrude68" cut 1 faces at (-99.386, -64.5486, -88.6475) along direction (-1, 0, 0) blind 33 on bodies 17 bodies 3 16 17
extrude "Extrude69" cut 3 faces at (-113.8527, -66.6686, -75.3142) (-125.7666, -66.6686, -75.3142) (-98.6194, -66.6686, -75.3142) along direction (0, 0, 1) blind 0.6 on bodies 3 16 17 bodies 3 16 17
extrude "Extrude70" add 3 faces at (-125.7666, -64.5486, -95.3142) (-113.8527, -64.5486, -95.3142) (-96.5027, -64.5486, -95.3142) along direction (0, 0, 1) blind 0.6 on bodies 3 16 17 bodies 3 16 17
move_body "Move50" bodies 15 to x (1, 0, 0) y (0, 1, 0) z (0, 0, 1) at (119.2809, -2.8797, 29.3525)
move_body "Move51" bodies 15 to x (1, 0, 0) y (0, 1, 0) z (0, 0, 1) at (0, 0, -4.202)
move_body "Move52" bodies 4 to x (1, 0, 0) y (0, 1, 0) z (0, 0, 1) at (0, 0, -6.35)
extrude "Extrude71" cut 1 faces at (61.916, -83.9013, -107.8386) along direction (0, 1, 0) blind 0.27 on bodies 5 bodies 5
extrude "Extrude72" cut 1 faces at (53.5408, -91.3613, -107.8386) along direction (0, -1, 0) blind 0.27 on bodies 5 bodies 5
move_face "MoveFace2" by (0, -0.499, 0) 1 faces at (13.6246, 20.4968, -105.7219) on bodies 5
move_face "MoveFace3" by (-0.298, 0, 0) 1 faces at (13.6246, 19.9978, -105.7219) on bodies 5
move_face "MoveFace4" by (-0.292, 0, 0) 1 faces at (13.6246, 19.9978, -105.7219) on bodies 5
move_body "Move53" bodies 5 to x (1, 0, 0) y (0, 1, 0) z (0, 0, 1) at (-0.292, 0, 0)
move_body "Move54" bodies 5 to x (1, 0, 0) y (0, 1, 0) z (0, 0, 1) at (0, 0.045, 0)
extrude "Extrude73" add 1 faces at (-43.3341, -149.4582, -105.7219) along direction (0, -1, 0) blind 0.544 on bodies 5 bodies 5 4 7 15 16 17 3
move_body "Move55" bodies 1 2 4 5 7 15 16 17 14 to x (-1, 0, 0) y (0, 1, 0) z (0, 0, -1) at (26.7765, 79.2164, 5.5754)
copy_body "Body->Comp2" bodies 14 removing the originals makes body 18 in component "Hand_R"
extrude "Extrude74" add 1 faces at (-68.9902, -9.667, 145.3436) along direction (0, 0, -1) blind 0.768 on bodies 5 bodies 5
extrude "Extrude75" cut 1 faces at (-26.4723, -4.37, 111.2973) along direction (0, -1, 0) blind 10 on bodies 5 bodies 5
extrude "Extrude76" add 1 faces at (-26.4723, -4.37, 111.2973) along direction (0, -1, 0) blind 10 on bodies 5 bodies 5
move_face "OffsetFaces1" offset 11.5 1 faces at (24.3636, -66.5503, 63.4676) on bodies 5
component "Hand_R" placed x (1, 0, 0) y (0, 1, 0) z (0, 0, 1) at (0, 0, 0)
named bodies: "Arduino", "Breadboard", "Exterior", "Roof (part of exterior)", "Arduino stand", "Servo stand", "Servo shelf", "Hand_R", "Hand_L"
